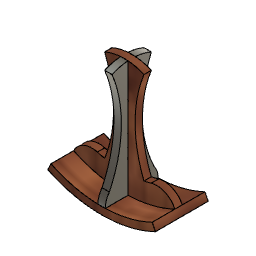
Stempel v5 (Autodesk Fusion 360 design; units mm, degrees)
Autodesk Fusion 360 part; units mm, degrees
note: some values were not read from the file. Chosen so that the rebuilt part matches the saved one: that a step has no effect.
sketch "Sketch1" plane through (0, 0, 0) normal (0, 1, 0) x (1, 0, 0)
  arc A0 (21.9089, -5) -> (-21.9089, -5) centre (0, -50.5) ccw
  line L0 (-21.9089, -5) -> (0, -50.5) construction
  line L1 (0, -50.5) -> (21.9089, -5) construction
  arc A1 (22.8937, -2.9548) -> (-22.8937, -2.9548) centre (0, -50.5) ccw
  line L2 (-22.8937, -2.9548) -> (-21.9089, -5)
  line L3 (21.9089, -5) -> (22.8937, -2.9548)
  arc A2 (20.6074, -7.703) -> (-20.6074, -7.703) centre (0, -50.5) ccw
  arc A3 (-20.6074, -7.703) -> (-10.9673, -12.0329) centre (-13.2164, -4.1441) ccw
  arc A4 (-8, -48.8303) -> (0, -50.5) centre (0, -30.5) ccw
  arc A5 (-8, -11.3082) -> (-10.9673, -12.0329) centre (0, -50.5) ccw
  arc A6 (-8, -48.8303) -> (-8, -11.3082) centre (-54.8857, -30.0692) ccw
  line L4 (0, -50.5) -> (-19.4173, 21.9662) construction
  line L5 (0, -50.5) -> (75.0683, -50.5) construction
  line L6 (3.8637, -49.4647) -> (-15.5536, 23.0015) construction
  line L7 (-3.8637, -51.5353) -> (-23.281, 20.931) construction
  line L8 (-16.893, -2.9093) -> (-16.1139, -5.8168)
  line L9 (-8.3865, -3.7462) -> (-9.1656, -0.8387)
  line L10 (0, -50.5) -> (0, 0) construction
  line L11 (8.3865, -3.7462) -> (9.1656, -0.8387)
  line L12 (16.893, -2.9093) -> (16.1139, -5.8168)
  arc A7 (10.9673, -12.0329) -> (20.6074, -7.703) centre (13.2164, -4.1441) ccw
  arc A8 (10.9673, -12.0329) -> (8, -11.3082) centre (0, -50.5) ccw
  arc A9 (8, -11.3082) -> (8, -48.8303) centre (54.8857, -30.0692) ccw
  arc A10 (0, -50.5) -> (8, -48.8303) centre (0, -30.5) ccw
  line L13 (-21.9089, -5) -> (-20.6074, -7.703)
  line L14 (20.6074, -7.703) -> (21.9089, -5)
  dimension "d1" = 5
  dimension "d4" = 50.5
  dimension "d5" = 2.27
  dimension "d6" = -3
  dimension "d7" = 20
  dimension "d8" = 50.5
  dimension "d9" = 8
  dimension "d10" = 8.2031
  dimension "d11" = 8
  dimension "d12" = 105
  dimension "d13" = 4
  dimension "d14" = -4
  constraint coincident L10.end A0
  constraint coincident A0.centre L0.end
  constraint vertical L10.end A0.centre
  constraint horizontal A0.end A0.start
  constraint parallel L0 L2
  constraint parallel L1 L3
  constraint tangent L0 A3
  constraint tangent A3 A5
  constraint tangent A4 A5
  constraint vertical L10.end A4.centre
  constraint horizontal L5
  constraint coincident A0 L8.start
  constraint coincident L7 L8.start
  constraint coincident A2 L8.end
  constraint coincident L7 L8.end
  constraint coincident A2 L9.start
  constraint coincident L6 L9.start
  constraint coincident A0 L9.end
  constraint coincident L6 L9.end
  constraint coincident L10.end origin
  constraint symmetric A2.end L10 A2.start
  constraint symmetric A3.end L10 A7.start
  constraint symmetric A3 L10 A7
  constraint symmetric A0.centre L10 L0.end
  constraint symmetric A4.start L10 A9.end
  constraint symmetric A4 L10 A10
  constraint symmetric A5.start L10 A8.end
  constraint symmetric A5 L10 A8
  constraint symmetric A6 L10 A9
  constraint symmetric L8.start L10 L12.start
  constraint symmetric L8.end L10 L12.end
  constraint symmetric L9.start L10 L11.start
  constraint symmetric L9.end L10 L11.end
  measures "d1" vertical distance of L10.end A0.end
  measures "d4" radius of A0
  measures "d7" radius of A4
  measures "d8" radius of A6
  measures "d9" horizontal distance of L10.end A5.start
  measures "d10" radius of A3
  measures "d11" horizontal distance of A4.start A0.centre
  measures "d12" angle of L4 L5
extrude "Extrude1" add sketch "Sketch1" along normal mid plane 3 contours A0 A2 L11 L12 | A2 A3 A4 A5 A6 A7 A8 A9 A10 | A0 A2 L8 L9 makes body 1
extrude "Extrude2" add sketch "Sketch1" along normal mid plane 21.5 separate body contours A0 A2 L12 L14 | A0 A2 L11 L12 | A0 A2 L9 L11 | A0 A2 L8 L9 | A0 A2 L8 L13 makes body 2
extrude "Extrude3" add sketch "Sketch1" along normal mid plane 3 separate body contours A0 A2 L11 L12 | A0 A2 L8 L9 makes body 3 at (-12.7232, 0.5, 4.7357) makes body 4 at (15.274, -0.5, 5.5227)
combine "Combine1" operation cut target body 2 tool bodies 3 4
sketch "Sketch2" plane through (0, -1.5, 0) normal (0, -1, 0) x (1, 0, 0)
  arc A0 (8, 48.8303) -> (-8, 48.8303) centre (0, 30.5) ccw
  arc A1 (-8, 11.3082) -> (-8, 48.8303) centre (-54.8857, 30.0692) ccw
  arc A2 (-10.9673, 12.0329) -> (-8, 11.3082) centre (0, 50.5) ccw
  arc A3 (-10.9673, 12.0329) -> (-20.6074, 7.703) centre (-13.2164, 4.1441) ccw
  arc A4 (-20.6074, 7.703) -> (-16.1139, 5.8168) centre (0, 50.5) ccw
  line L0 (-16.1139, 5.8168) -> (-16.893, 2.9093)
  arc A5 (-16.893, 2.9093) -> (-9.1656, 0.8387) centre (0, 50.5) ccw
  line L1 (-9.1656, 0.8387) -> (-8.3865, 3.7462)
  arc A6 (-8.3865, 3.7462) -> (8.3865, 3.7462) centre (0, 50.5) ccw
  line L2 (8.3865, 3.7462) -> (9.1656, 0.8387)
  arc A7 (9.1656, 0.8387) -> (16.893, 2.9093) centre (0, 50.5) ccw
  line L3 (16.893, 2.9093) -> (16.1139, 5.8168)
  arc A8 (16.1139, 5.8168) -> (20.6074, 7.703) centre (0, 50.5) ccw
  arc A9 (20.6074, 7.703) -> (10.9673, 12.0329) centre (13.2164, 4.1441) ccw
  arc A10 (8, 11.3082) -> (10.9673, 12.0329) centre (0, 50.5) ccw
  arc A11 (8, 48.8303) -> (8, 11.3082) centre (54.8857, 30.0692) ccw
  line L4 (0, 50.5) -> (0, 0) construction
  line L5 (-1.5, 25) -> (1.5, 25)
  line L6 (1.5, -1) -> (-1.5, -1)
  line L7 (-1.5, 35) -> (1.5, 35)
  line L8 (1.5, 35) -> (1.5, 45)
  line L9 (1.5, 45) -> (-1.5, 45)
  line L10 (-1.5, 45) -> (-1.5, 35)
  line L11 (-1.5, 17) -> (-1.3, 15)
  line L12 (-1.3, 15) -> (-1.5, 15)
  line L13 (1.5, 15) -> (1.3, 15)
  line L14 (1.3, 15) -> (1.5, 17)
  line L15 (-1.5, -1) -> (-1.5, 15)
  line L16 (-1.5, 17) -> (-1.5, 25)
  line L17 (-1.5, 15) -> (-1.5, 17)
  line L18 (1.5, 25) -> (1.5, 17)
  line L19 (1.5, 15) -> (1.5, -1)
  line L20 (1.5, 17) -> (1.5, 15)
  dimension "d21" = 3
  dimension "d22" = 1.5
  dimension "d23" = 1
  dimension "d24" = 26
  dimension "d25" = 10
  dimension "d26" = 10
  dimension "d27" = 10
  dimension "d28" = 10
  dimension "d29" = 0.2
  dimension "d30" = 0.2
  dimension "d31" = 2
  dimension "d32" = 2
  constraint coincident A2.centre A4.centre
  constraint coincident L4.end origin
  constraint horizontal L5
  constraint vertical L18
  constraint horizontal L6
  constraint vertical L15
  constraint horizontal L7
  constraint vertical L8
  constraint horizontal L9
  constraint vertical L10
  constraint coincident L11.start L15
  constraint perpendicular L12 L15
  constraint coincident L13.start L18
  constraint perpendicular L13 L18
  constraint vertical L19
  constraint vertical L16
  constraint coincident L5.start L10
  constraint coincident L5.end L8
  measures "d21" distance of L6.start L6.end
  measures "d22" horizontal distance of L6.start L4.end
  measures "d23" distance of L4.end L6
  measures "d24" distance of L5.end L6.start
  measures "d25" distance of L5.start L7.start
  measures "d26" distance of L7.start L9.end
  measures "d27" vertical distance of L5.start L11.end
  measures "d28" distance of L5.end L13
  measures "d29" distance of L11.end L12.end
  measures "d30" distance of L13.start L13.end
  measures "d31" distance of L11.start L12
  measures "d32" distance of L13 L14.end
extrude "Extrude4" cut sketch "Sketch2" against normal through all contours A6 L5 L11 L12 L13 L14 L15 L16 L18 L19 | L7 L8 L9 L10 bodies 1
sketch "Sketch3" plane through (0, 0, 0) normal (1, 0, 0) x (0, 1, 0)
  line L0 (1.5, 48.8303) -> (1.5, 50.5)
  line L1 (1.5, 48.8303) -> (1.5, 11.3082)
  line L2 (10.75, 7.703) -> (10.75, 3)
  line L3 (10.75, 0) -> (10.75, 5)
  line L4 (-1.5, 11.3082) -> (-1.5, 48.8303)
  line L5 (-1.5, 50.5) -> (-1.5, 48.8303)
  line L6 (-10.75, 3) -> (-10.75, 7.703)
  line L7 (1.5, 7.703) -> (1.5, 12.3473)
  line L8 (10.75, 0) -> (10.75, 3) construction
  arc A0 (10.75, 3) -> (9.0723, 7.9699) centre (2.55, 3) ccw
  arc A1 (8, 48.8303) -> (0, 50.5) centre (0, 30.5) ccw
  arc A2 (8, 48.8303) -> (9.0723, 7.9699) centre (54.7, 29.6116) ccw
  line L9 (10.75, 3) -> (0, 3)
  line L10 (8.75, 0) -> (8.75, 3)
  line L11 (2.75, 0) -> (2.75, 3)
  line L12 (8.75, 0) -> (2.75, 0)
  line L13 (0, 50.5) -> (0, 3) construction
  arc A3 (0, 50.5) -> (-8, 48.8303) centre (0, 30.5) ccw
  arc A4 (-9.0723, 7.9699) -> (-8, 48.8303) centre (-54.7, 29.6116) ccw
  arc A5 (-9.0723, 7.9699) -> (-10.75, 3) centre (-2.55, 3) ccw
  line L14 (-10.75, 3) -> (0, 3)
  line L15 (-8.75, 0) -> (-8.75, 3)
  line L16 (-8.75, 0) -> (-2.75, 0)
  line L17 (-2.75, 0) -> (-2.75, 3)
  dimension "d34" = 8
  dimension "d35" = 20
  dimension "d36" = 50.5
  dimension "d37" = 54.7
  dimension "d38" = 8.2
  dimension "d39" = -2
  dimension "d40" = -8
  constraint coincident L3.start L8.start
  constraint coincident L2.end L8.end
  constraint tangent L2 A0
  constraint vertical origin A1.centre
  constraint vertical A1.end A1.centre
  constraint horizontal L5.start A1.end
  constraint perpendicular L2 L9
  constraint perpendicular L11 L12
  constraint perpendicular L9 L13
  constraint symmetric L2.end L13 L6.start
  constraint symmetric A0.end L13 A4.start
  constraint symmetric A0 L13 A5
  constraint symmetric A1.end L13 A3.start
  constraint symmetric A1.start L13 A3.end
  constraint symmetric A1 L13 A3
  constraint symmetric A2 L13 A4
  constraint symmetric L9.end L13 L14.end
  constraint symmetric L10.start L13 L15.start
  constraint symmetric L10.end L13 L15.end
  constraint symmetric L11.start L13 L16.end
  constraint symmetric L11.end L13 L17.end
  measures "d34" horizontal distance of origin A1.start
  measures "d35" radius of A1
  measures "d36" radius of A2
  measures "d37" horizontal distance of origin A2.centre
  measures "d38" radius of A0
extrude "Extrude5" add sketch "Sketch3" along normal mid plane 3 separate body makes body 5
sketch "Sketch4" plane through (-1.5, 0, 0) normal (-1, 0, 0) x (0, -1, 0)
  line L0 (2.75, 0) -> (8.75, 0)
  line L1 (8.75, 0) -> (8.75, 3)
  line L2 (8.75, 3) -> (10.75, 3)
  arc A0 (10.75, 3) -> (9.0723, 7.9699) centre (2.55, 3) ccw
  arc A1 (8, 48.8303) -> (9.0723, 7.9699) centre (54.7, 29.6116) ccw
  arc A2 (8, 48.8303) -> (-8, 48.8303) centre (0, 30.5) ccw
  arc A3 (-9.0723, 7.9699) -> (-8, 48.8303) centre (-54.7, 29.6116) ccw
  arc A4 (-9.0723, 7.9699) -> (-10.75, 3) centre (-2.55, 3) ccw
  line L3 (-10.75, 3) -> (-8.75, 3)
  line L4 (-8.75, 3) -> (-8.75, 0)
  line L5 (-8.75, 0) -> (-2.75, 0)
  line L6 (-2.75, 0) -> (-2.75, 3)
  line L7 (-2.75, 3) -> (2.75, 3)
  line L8 (2.75, 3) -> (2.75, 0)
  line L9 (1.5, 45) -> (1.5, 35)
  line L10 (1.5, 25) -> (-1.5, 25)
  line L11 (-1.5, 25) -> (-1.5, 52.5)
  line L12 (-1.5, 52.5) -> (1.5, 52.5)
  line L13 (1.5, 52.5) -> (1.5, 25)
  line L14 (1.5, 35) -> (1.3, 35)
  line L15 (1.3, 35) -> (1.5, 37)
  line L16 (-1.5, 35) -> (-1.3, 35)
  line L17 (-1.3, 35) -> (-1.5, 37)
  line L18 (1.5, 15) -> (-1.5, 15)
  line L19 (-1.5, 15) -> (-1.5, 20)
  line L20 (-1.5, 20) -> (1.5, 20)
  line L21 (1.5, 20) -> (1.5, 15)
  point P0 (1.5, 25)
  point P1 (1.5, 15)
  dimension "d43" = 3
  dimension "d44" = 27.5
  dimension "d45" = 3
  dimension "d46" = 5
  dimension "d47" = 0.2
  dimension "d48" = 0.2
  dimension "d49" = 2
  dimension "d50" = 2
  constraint horizontal L10
  constraint vertical L11
  constraint horizontal L12
  constraint vertical L13
  constraint coincident P0 L10.start
  constraint coincident L9.end L14.start
  constraint perpendicular L9 L14
  constraint coincident L9 L15.end
  constraint coincident L11 L16.start
  constraint perpendicular L11 L16
  constraint coincident L11 L17.end
  constraint horizontal L18
  constraint vertical L19
  constraint horizontal L20
  constraint vertical L21
  constraint coincident P1 L18.start
  constraint coincident L14 L16.end
  measures "d43" distance of P0 L10.end
  measures "d44" distance of P0 L12.end
  measures "d45" distance of P1 L18.end
  measures "d46" distance of P1 L20.end
  measures "d47" distance of L9.end L14.end
  measures "d48" distance of L16.start L16.end
  measures "d49" distance of L14 L15.end
  measures "d50" distance of L16 L17.end
extrude "Extrude6" cut sketch "Sketch4" against normal blind 4.024 contours A2 L9 L10 L11 L13 L14 L15 L16 L17 | A2 L11 L12 L13 | L18 L19 L20 L21 bodies 5
sketch "Sketch5" plane through (0, -8.75, 0) normal (0, -1, 0) x (1, 0, 0)
  line L0 (-1.5, 0) -> (1.5, 0)
  line L1 (1.5, 0) -> (1.5, 3)
  line L2 (1.5, 3) -> (-1.5, 3)
  line L3 (-1.5, 3) -> (-1.5, 0)
  arc A0 (-21.9089, 5) -> (21.9089, 5) centre (0, 50.5) ccw
  line L4 (-2.0005, 0.0396) -> (-2.0005, -1.4666)
  line L5 (-2.0005, -1.4666) -> (3.2426, -1.4666)
  line L6 (3.2426, -1.4666) -> (3.2426, 0.1042)
  constraint coincident A0 L4.start
  constraint vertical L4
  constraint perpendicular L4 L5
  constraint coincident A0 L6.end
  constraint perpendicular L5 L6
extrude "Extrude7" cut sketch "Sketch5" against normal through all contours L0 L3 A0 | L0 L1 L3 A0 L4 L5 L6 | L0 L1 A0 bodies 5
sketch "Sketch6" plane through (0, 0, 3) normal (0, 0, -1) x (1, 0, 0)
  line L0 (-1.5, 8.75) -> (1.5, 8.75)
  line L1 (1.5, 8.75) -> (1.5, 10.75)
  line L2 (1.5, 10.75) -> (-1.5, 10.75)
  line L3 (-1.5, 10.75) -> (-1.5, 8.75)
  line L4 (-1.5, 2.75) -> (1.5, 2.75)
  line L5 (1.5, 2.75) -> (1.5, 8.75)
  line L6 (1.5, 8.75) -> (-1.5, 8.75)
  line L7 (-1.5, 8.75) -> (-1.5, 2.75)
  line L8 (-1.5, -8.75) -> (1.5, -8.75)
  line L9 (1.5, -8.75) -> (1.5, -2.75)
  line L10 (1.5, -2.75) -> (-1.5, -2.75)
  line L11 (-1.5, -2.75) -> (-1.5, -8.75)
extrude "Extrude8" cut sketch "Sketch6" along normal mid plane 7.316 contours L0 L4 L5 L6 L7 | L8 L9 L10 L11 bodies 2
step "ConvertToSheetMetal1" [no effect]
sketch "Sketch7" plane through (0, -1.5, 0) normal (0, -1, 0) x (1, 0, 0)
  line L0 (-1.5, 3.0237) -> (-1.5, 15)
  line L1 (-1.5, 15) -> (-1.3, 15)
  line L2 (-1.3, 15) -> (-1.5, 17)
  line L3 (-1.5, 17) -> (-1.5, 25)
  line L4 (-1.5, 25) -> (1.5, 25)
  line L5 (1.5, 25) -> (1.5, 17)
  line L6 (1.5, 17) -> (1.3, 15)
  line L7 (1.3, 15) -> (1.5, 15)
  line L8 (1.5, 15) -> (1.5, 3.0237)
  arc A0 (1.5, 3.0237) -> (8.3865, 3.7462) centre (0, 50.5) ccw
  line L9 (8.3865, 3.7462) -> (9.1656, 0.8387)
  arc A1 (9.1656, 0.8387) -> (16.893, 2.9093) centre (0, 50.5) ccw
  line L10 (16.893, 2.9093) -> (16.1139, 5.8168)
  arc A2 (16.1139, 5.8168) -> (20.6074, 7.703) centre (0, 50.5) ccw
  arc A3 (20.6074, 7.703) -> (10.9673, 12.0329) centre (13.2164, 4.1441) ccw
  arc A4 (8, 11.3082) -> (10.9673, 12.0329) centre (0, 50.5) ccw
  arc A5 (8, 48.8303) -> (8, 11.3082) centre (54.8857, 30.0692) ccw
  arc A6 (8, 48.8303) -> (-8, 48.8303) centre (0, 30.5) ccw
  arc A7 (-8, 11.3082) -> (-8, 48.8303) centre (-54.8857, 30.0692) ccw
  arc A8 (-10.9673, 12.0329) -> (-8, 11.3082) centre (0, 50.5) ccw
  arc A9 (-10.9673, 12.0329) -> (-20.6074, 7.703) centre (-13.2164, 4.1441) ccw
  arc A10 (-20.6074, 7.703) -> (-16.1139, 5.8168) centre (0, 50.5) ccw
  line L11 (-16.1139, 5.8168) -> (-16.893, 2.9093)
  arc A11 (-16.893, 2.9093) -> (-9.1656, 0.8387) centre (0, 50.5) ccw
  line L12 (-9.1656, 0.8387) -> (-8.3865, 3.7462)
  arc A12 (-8.3865, 3.7462) -> (-1.5, 3.0237) centre (0, 50.5) ccw
  line L13 (-1.5, 45) -> (1.5, 45)
  line L14 (1.5, 45) -> (1.5, 35)
  line L15 (1.5, 35) -> (-1.5, 35)
  line L16 (-1.5, 35) -> (-1.5, 45)
sketch "Sketch8" plane through (1.5, 0, 0) normal (1, 0, 0) x (0, 1, 0)
  line L0 (2.75, 0.0223) -> (8.75, 0.0223)
  line L1 (8.75, 0.0223) -> (8.75, 3)
  line L2 (8.75, 3) -> (10.75, 3)
  arc A0 (10.75, 3) -> (9.0723, 7.9699) centre (2.55, 3) ccw
  arc A1 (8, 48.8303) -> (9.0723, 7.9699) centre (54.7, 29.6116) ccw
  arc A2 (8, 48.8303) -> (1.5, 50.4437) centre (0, 30.5) ccw
  line L3 (1.5, 50.4437) -> (1.5, 37)
  line L4 (1.5, 37) -> (1.3, 35)
  line L5 (1.3, 35) -> (1.5, 35)
  line L6 (1.5, 35) -> (1.5, 25)
  line L7 (1.5, 25) -> (-1.5, 25)
  line L8 (-1.5, 25) -> (-1.5, 35)
  line L9 (-1.5, 35) -> (-1.3, 35)
  line L10 (-1.3, 35) -> (-1.5, 37)
  line L11 (-1.5, 37) -> (-1.5, 50.4437)
  arc A3 (-1.5, 50.4437) -> (-8, 48.8303) centre (0, 30.5) ccw
  arc A4 (-9.0723, 7.9699) -> (-8, 48.8303) centre (-54.7, 29.6116) ccw
  arc A5 (-9.0723, 7.9699) -> (-10.75, 3) centre (-2.55, 3) ccw
  line L12 (-10.75, 3) -> (-8.75, 3)
  line L13 (-8.75, 3) -> (-8.75, 0.0223)
  line L14 (-8.75, 0.0223) -> (-2.75, 0.0223)
  line L15 (-2.75, 0.0223) -> (-2.75, 3)
  line L16 (-2.75, 3) -> (2.75, 3)
  line L17 (2.75, 3) -> (2.75, 0.0223)
  line L18 (1.5, 20) -> (1.5, 15)
  line L19 (1.5, 15) -> (-1.5, 15)
  line L20 (-1.5, 15) -> (-1.5, 20)
  line L21 (-1.5, 20) -> (1.5, 20)
component "stempel" placed x (1, 0, 0) y (0, 1, 0) z (0, 0, 1) at (0, 0, 0)
equation "d37 = 50.5 mm + 4.2 mm"
